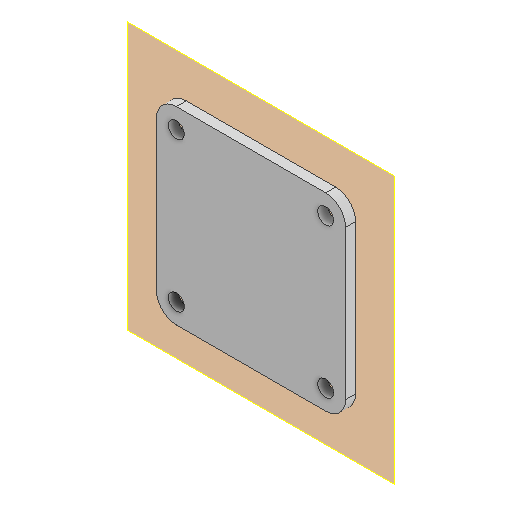
# Autodesk Inventor part: 20_Cube_Insert_SEEED_Xiao_Sense_Camera_backplate
Saved by Autodesk Inventor 2022 (Build 260153000, 153)
## iProperties
Created: 2023-04-27
Part Number: 20_Cube_Insert_SEEED_Xiao_Sense_Camera_backplate
Material: Generisch
Document SubType Name: Modeling
Designer: diederichbenedict
Density: 1 g/cm^3
Appearance: Vorgabe
Author: diederichbenedict
Autodesk Inventor part; units mm, degrees
ref_plane "YZ Plane" through (0, 0, 0) normal (1, 0, 0) x (0, 1, 0)
ref_plane "XZ Plane" through (0, 0, 0) normal (0, 1, 0) x (-1, 0, 0)
ref_plane "XY Plane" through (0, 0, 0) normal (0, 0, 1) x (1, 0, 0)
ref_plane "Arbeitsebene1" through (0, 0, 0) normal (0, 0, 1) x (1, 0, 0)
sketch "Skizze1" plane through (0, 0, 0) normal (0, 0, 1) x (1, 0, 0)
  line L0 (14.5712, 11.3758) -> (14.5712, 4.0068) projected
  line L1 (13.3638, -15.5) -> (13.3638, 1.7) projected
  arc A0 (14.5712, 4.0068) -> (13.3638, 1.7) centre (16.1712, 1.7) ccw projected
  line L2 (8.0712, 15) -> (38.0712, 15)
  line L3 (38.0712, 15) -> (38.0712, -15)
  line L4 (38.0712, -15) -> (8.0712, -15)
  line L5 (8.0712, -15) -> (8.0712, 15)
  line L6 (38.0712, 19) -> (8.0712, 19)
  line L7 (4.0712, 15) -> (4.0712, -15)
  line L8 (8.0712, -19) -> (38.0712, -19)
  line L9 (42.0712, -15) -> (42.0712, 15)
  arc A1 (8.0712, 19) -> (4.0712, 15) centre (8.0712, 15) ccw
  arc A2 (42.0712, 15) -> (38.0712, 19) centre (38.0712, 15) ccw
  arc A3 (38.0712, -19) -> (42.0712, -15) centre (38.0712, -15) ccw
  arc A4 (4.0712, -15) -> (8.0712, -19) centre (8.0712, -15) ccw
  line L10 (10.5793, 11.3758) -> (14.5712, 11.3758) projected
  line L11 (36.5793, 10.3758) -> (36.5793, -24.4) projected
  arc A5 (36.5793, 10.3758) -> (35.5793, 11.3758) centre (35.5793, 10.3758) ccw projected
  line L12 (9.5793, -24.4) -> (9.5793, 10.3758) projected
  line L13 (36.5793, -24.4) -> (9.5793, -24.4) projected
  line L14 (31.5712, 11.3758) -> (35.5793, 11.3758) projected
  line L15 (31.5712, 4.0068) -> (31.5712, 11.3758) projected
  arc A6 (10.5793, 11.3758) -> (9.5793, 10.3758) centre (10.5793, 10.3758) ccw projected
  arc A7 (32.7786, 1.7) -> (31.5712, 4.0068) centre (29.9712, 1.7) ccw projected
  line L16 (32.7786, 1.7) -> (32.7786, -15.5) projected
  arc A8 (29.9712, -18.3074) -> (32.7786, -15.5) centre (29.9712, -15.5) ccw projected
  line L17 (29.9712, -18.3074) -> (16.1712, -18.3074) projected
  arc A9 (13.3638, -15.5) -> (16.1712, -18.3074) centre (16.1712, -15.5) ccw projected
  point P0 (0, 0)
  dimension "d0" = 4
  dimension "d1" = 4
  constraints: 16 end point, 8 point on circle, 8 tangent, 4 centre point, 4 parallel, 3 equal radius, 2 perpendicular, 1 horizontal, 3 other
  measures "d0" distance between parallel lines of L2 L6
  measures "d1" radius of A1
extrude "Extrusion1" add sketch "Skizze1" along normal blind 2 contours L10 A6 L12 L4 L5 L2 L3 L11 A5 L14 L15 A7 L16 L1 A0 L0 | L0 A0 L1 L4 L12 A6 L10 | L4 L16 A8 L17 A9 L1 | L1 A9 L17 A8 L16 L4 L11 L8 L12 | L12 L8 A4 L7 A1 L6 A2 L9 A3 L11 L4 L3 L2 L5 | L16 A7 L15 L14 A5 L11 L4
ref_plane "Arbeitsebene2" through (0, 0, 0) normal (0, 0, 1) x (1, 0, 0)
sketch "Skizze2" plane through (0, 0, 2) normal (0, 0, 1) x (1, 0, 0)
  arc A0 (8.0712, 19) -> (4.0712, 15) centre (8.0712, 15) ccw projected
  line L0 (4.0712, 15) -> (4.0712, -15) projected
  arc A1 (4.0712, -15) -> (8.0712, -19) centre (8.0712, -15) ccw projected
  line L1 (8.0712, -19) -> (38.0712, -19) projected
  arc A2 (38.0712, -19) -> (42.0712, -15) centre (38.0712, -15) ccw projected
  line L2 (42.0712, -15) -> (42.0712, 15) projected
  arc A3 (42.0712, 15) -> (38.0712, 19) centre (38.0712, 15) ccw projected
  line L3 (38.0712, 19) -> (8.0712, 19) projected
  circle A4 centre (8.0712, 15) radius 1.4 projected
  circle A5 centre (38.0712, 15) radius 1.4 projected
  circle A6 centre (38.0712, -15) radius 1.4 projected
  circle A7 centre (8.0712, -15) radius 1.4 projected
  point P0 (0, 0)
hole "Bohrung1" at (8.0712, 15, 2) at (8.0712, -15, 2) at (38.0712, -15, 2) at (38.0712, 15, 2) direction (0, 0, -1) diameter 3.2 end through all
